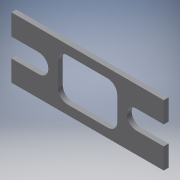
# Autodesk Inventor part: headplate_largerCenter
Saved by Autodesk Inventor 2016 (Build 200138000, 138)
## iProperties
Created: 2011-10-05
Part Number: headplate_largerCenter
Material: Generic
Document SubType Name: Modeling
Designer: charvey
Density: 1 g/cm^3
Appearance: Default
Author: charvey
Autodesk Inventor part; units mm, degrees
ref_plane "YZ Plane" through (0, 0, 0) normal (1, 0, 0) x (0, 1, 0)
ref_plane "XZ Plane" through (0, 0, 0) normal (0, 1, 0) x (-1, 0, 0)
sketch "Sketch1" plane through (0, 0, 0) normal (0, 0, 1) x (1, 0, 0)
  line L0 (-12.7, 5.08) -> (12.7, 5.08)
  line L1 (12.7, 5.08) -> (12.7, -5.08)
  line L2 (12.7, -5.08) -> (-12.7, -5.08)
  line L3 (-12.7, -5.08) -> (-12.7, 5.08)
  point P0 (0, 0)
  point P1 (0, 5.08)
  point P2 (-12.7, 0)
  dimension "d0" = 25.4
  dimension "d1" = 10.16
  constraints: 8 end point, 2 midpoint, 2 parallel, 1 horizontal, 1 horizontal alignment, 1 perpendicular, 1 vertical alignment
  measures "d0" distance between parallel lines of L1 L3
  measures "d1" distance between parallel lines of L2 L0
extrude "Extrusion1" add sketch "Sketch1" along normal blind 0.8128
ref_plane "Work Plane1" through (0, 0, 13.5128) normal (0, 0, 1) x (1, 0, 0)
sketch "Sketch2" plane through (0, 0, 13.5128) normal (0, 0, 1) x (1, 0, 0)
  line L0 (12.7, 5.08) -> (12.7, -5.08) projected
  line L1 (-12.7, 5.08) -> (12.7, 5.08) projected
  line L2 (-12.7, -5.08) -> (-12.7, 5.08) projected
  line L3 (12.7, -5.08) -> (-12.7, -5.08) projected
  line L4 (-3.3655, 3.556) -> (3.3655, 3.556)
  line L5 (-3.3655, -3.556) -> (3.3655, -3.556)
  line L6 (-4.953, 1.9685) -> (-4.953, -1.9685)
  line L7 (4.953, 1.9685) -> (4.953, -1.9685)
  arc A0 (-3.3655, 3.556) -> (-4.953, 1.9685) centre (-3.3655, 1.9685) ccw
  arc A1 (-4.953, -1.9685) -> (-3.3655, -3.556) centre (-3.3655, -1.9685) ccw
  arc A2 (3.3655, -3.556) -> (4.953, -1.9685) centre (3.3655, -1.9685) ccw
  arc A3 (4.953, 1.9685) -> (3.3655, 3.556) centre (3.3655, 1.9685) ccw
  point P0 (0, 0)
  point P1 (0, 3.556)
  point P2 (0, -3.556)
  point P3 (-4.953, 0)
  point P4 (4.953, 0)
  dimension "d5" = 6.731
  dimension "d6" = 6.731
  dimension "d7" = 3.937
  dimension "d8" = 3.937
  dimension "d9" = 4.953
  dimension "d10" = 4.953
  dimension "d11" = 3.556
  dimension "d12" = 3.556
  dimension "d13" = 1.5875
  dimension "d14" = 1.5875
  dimension "d15" = 1.5875
  dimension "d16" = 1.5875
  constraints: 8 end point, 8 point on circle, 4 centre point, 4 midpoint, 3 parallel, 2 horizontal alignment, 2 vertical alignment, 1 perpendicular
  measures "d5" distance of L4.end L4.start
  measures "d6" distance of L5.end L5.start
  measures "d7" distance of L6.end L6.start
  measures "d8" distance of L7.end L7.start
  measures "d9" distance of point (-4.953, 0) point (0, 0)
  measures "d10" distance of point (4.953, 0) point (0, 0)
  measures "d11" distance of point (0, 3.556) point (0, 0)
  measures "d12" distance of point (0, -3.556) point (0, 0)
  measures "d13" radius of A0
  measures "d14" radius of A1
  measures "d15" radius of A2
  measures "d16" radius of A3
extrude "Extrusion2" cut sketch "Sketch2" against normal blind 25.4 contours L4 A3 L7 A2 L5 A1 L6 A0
sketch "Sketch3" plane through (0, 0, 13.5128) normal (0, 0, 1) x (1, 0, 0)
  arc A0 (-3.3655, 3.556) -> (-4.953, 1.9685) centre (-3.3655, 1.9685) ccw projected
  line L0 (-3.3655, 3.556) -> (3.3655, 3.556) projected
  arc A1 (4.953, 1.9685) -> (3.3655, 3.556) centre (3.3655, 1.9685) ccw projected
  line L1 (4.953, 1.9685) -> (4.953, -1.9685) projected
  arc A2 (3.3655, -3.556) -> (4.953, -1.9685) centre (3.3655, -1.9685) ccw projected
  line L2 (3.3655, -3.556) -> (-3.3655, -3.556) projected
  arc A3 (-4.953, -1.9685) -> (-3.3655, -3.556) centre (-3.3655, -1.9685) ccw projected
  line L3 (-4.953, -1.9685) -> (-4.953, 1.9685) projected
  line L4 (12.7, 5.08) -> (12.7, -5.08) projected
  line L5 (-12.7, 5.08) -> (12.7, 5.08) projected
  line L6 (-12.7, -5.08) -> (-12.7, 5.08) projected
  line L7 (12.7, -5.08) -> (-12.7, -5.08) projected
  line L8 (-12.7, 1.5875) -> (-8.128, 1.5875)
  line L9 (-12.7, -1.5875) -> (-8.128, -1.5875)
  arc A4 (-8.128, -1.5875) -> (-8.128, 1.5875) centre (-8.128, 0) ccw
  point P0 (0, 0)
  dimension "d19" = 4.572
  dimension "d20" = 3.4925
  dimension "d21" = 4.572
  dimension "d22" = 3.175
  dimension "d24" = 1.5875
  constraints: 4 end point, 2 parallel, 2 point on circle, 2 point on line, 1 centre point
  measures "d19" distance of L8.start L8.end
  measures "d20" distance between parallel lines of L8 L5
  measures "d21" distance of L9.start L9.end
  measures "d22" distance between parallel lines of L8 L9
  measures "d24" radius of A4
extrude "Extrusion3" cut sketch "Sketch3" against normal blind 25.4 contours L8 A4 L9 L6
mirror "Mirror1" about plane through (0, 0, 0) normal (1, 0, 0) of "Extrusion3"
body "Solid1"
